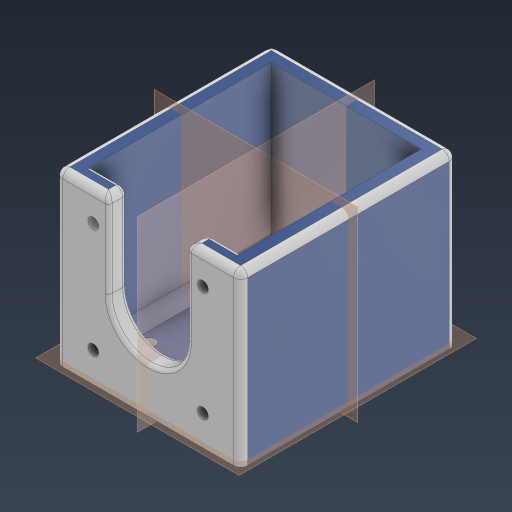
# Autodesk Inventor part: Крепление_мотора
Saved by Autodesk Inventor 2023.2 (Build 272271030, 271C)
## iProperties
Created: 2025-12-13
Part Number: Крепление_мотора
Material: Типовые
Document SubType Name: Modeling
Designer: Олег Коноваленко
Density: 1 g/cm^3
Appearance: По умолчанию
Author: Олег Коноваленко
Autodesk Inventor part; units mm, degrees
sketch "Эскиз1" plane through (0, 0, 0) normal (0, 1, 0) x (-1, 0, 0)
  line L0 (21.15, 25.5) -> (-21.15, 25.5)
  line L1 (-21.15, 25.5) -> (-21.15, -25.5)
  line L2 (-21.15, -25.5) -> (21.15, -25.5)
  line L3 (21.15, -25.5) -> (21.15, 25.5)
  line L4 (21.15, 25.5) -> (-21.15, -25.5) construction
  line L5 (-21.15, 25.5) -> (21.15, -25.5) construction
  point P0 (0, 0)
  dimension "d2" = 51
  dimension "d3" = 42.3
  constraints: 12 end point, 2 midpoint, 2 parallel, 1 horizontal, 1 perpendicular
  measures "d2" distance of L0.end L1.end
  measures "d3" distance of L1.end L2.end
extrude "Выдавливание1" add sketch "Эскиз1" along normal mid plane 2.85
sketch "Эскиз2" plane through (0, 1.425, 0) normal (0, 1, 0) x (1, 0, 0)
  line L0 (-21.15, -25.5) -> (-21.15, 25.5) projected
  line L1 (-21.15, 25.5) -> (-26.15, 25.5)
  line L2 (-26.15, 25.5) -> (-26.15, -25.5)
  line L3 (-26.15, -25.5) -> (-21.15, -25.5)
  line L4 (-21.15, -25.5) -> (-21.15, 25.5)
  point P0 (0, 0)
  dimension "d4" = 5
  constraints: 8 end point, 2 parallel, 1 horizontal, 1 perpendicular, 1 point on line
  measures "d4" distance of L0.end L1.end
extrude "Выдавливание2" add sketch "Эскиз2" along normal blind 45.15 and the other way blind 2.85
mirror "Зеркальное отражение1" about plane through (0, 0, 0) normal (1, 0, 0) of "Выдавливание2"
chamfer "Фаска1" distance 3.2 angle 45 2 edges at (-21.15, 1.425, 0) (21.15, 1.425, 0)
sketch "Эскиз3" plane through (0, 1.425, 0) normal (0, 1, 0) x (1, 0, 0)
  line L0 (-26.15, 25.5) -> (26.15, 25.5) projected
  line L1 (-26.15, 25.5) -> (26.15, 25.5)
  line L2 (26.15, 25.5) -> (26.15, 30.5)
  line L3 (26.15, 30.5) -> (-26.15, 30.5)
  line L4 (-26.15, 30.5) -> (-26.15, 25.5)
  point P0 (0, 0)
  dimension "d17" = 5
  constraints: 8 end point, 2 parallel, 1 horizontal, 1 perpendicular, 1 point on line
  measures "d17" distance of L3.end L0.start
extrude "Выдавливание3" add sketch "Эскиз3" along normal blind 45.15 and the other way blind 2.85
mirror "Зеркальное отражение2" about plane through (0, 0, 0) normal (0, 0, 1) of "Выдавливание3"
sketch "Эскиз7" plane through (-26.15, -1.425, 30.5) normal (0, 0, 1) x (1, 0, 0)
  circle A0 centre (26.15, 24) radius 11 projected
  circle A1 centre (26.15, 24) radius 11.2
  point P0 (26.15, 1.425)
  dimension "d22" = 22.4
  constraints: 1 centre point, 1 coincident
  measures "d22" diameter of A1
extrude "Выдавливание5" cut sketch "Эскиз7" against normal up to next contours A0 | A1
sketch "Эскиз8" plane through (-26.15, -1.425, 30.5) normal (0, 0, 1) x (1, 0, 0)
  circle A0 centre (26.15, 24) radius 11.2 projected
  line L0 (14.95, 24) -> (14.95, 48)
  line L1 (5, 48) -> (47.3, 48) projected
  line L2 (37.35, 24) -> (37.35, 48.1316)
  point P0 (26.15, 1.425)
  point P1 (37.35, 48)
  dimension "d23" = 22.4
  constraints: 4 end point, 2 perpendicular, 2 point on circle, 1 point on line
  measures "d23" distance between parallel lines of L2 L0
extrude "Выдавливание6" cut sketch "Эскиз8" against normal up to next contours A0 L0 L1 L2
fillet "Сопряжение1" radius 2 11 edges at (-11.2, 46.575, 28) (11.2, 46.575, 28) (-26.15, 46.575, 0) (-18.675, 46.575, 30.5) (18.675, 46.575, 30.5) (26.15, 46.575, 0) (0, 46.575, -30.5) (26.15, 22.575, 30.5) (-26.15, 22.575, 30.5) (-26.15, 22.575, -30.5) (26.15, 22.575, -30.5)
fillet "Сопряжение2" radius 1 12 edges at (0, 11.375, 25.5) (11.2, 33.575, 25.5) (11.7858, 45.9892, 25.5) (17.175, 46.575, 25.5) (-11.7858, 45.9892, 25.5) (-17.175, 46.575, 25.5) (-11.2, 33.575, 25.5) (-11.7858, 45.9892, 29.9142) (0, 11.375, 30.5) (11.2, 33.575, 30.5) (11.7858, 45.9892, 29.9142) (-11.2, 33.575, 30.5)
sketch "Эскиз9" plane through (-24.15, -1.425, 30.5) normal (0, 0, 1) x (1, 0, 0)
  circle A0 centre (8.65, 39.5) radius 1.5
  circle A1 centre (39.65, 39.5) radius 1.5
  circle A2 centre (39.65, 8.5) radius 1.5
  circle A3 centre (8.65, 8.5) radius 1.5
  line L0 (8.65, 39.5) -> (39.65, 39.5) construction
  line L1 (39.65, 39.5) -> (39.65, 8.5) construction
  line L2 (39.65, 8.5) -> (8.65, 8.5) construction
  line L3 (8.65, 8.5) -> (8.65, 39.5) construction
  arc A4 (12.95, 24) -> (35.35, 24) centre (24.15, 24) ccw projected
  line L4 (8.65, 39.5) -> (39.65, 8.5) construction
  line L5 (39.65, 39.5) -> (8.65, 8.5) construction
  line L6 (24.15, 62.1506) -> (24.15, -10.3584) projected
  point P0 (24.15, 1.425)
  point P1 (24.15, 24)
  point P2 (24.15, 24)
  dimension "d28" = 3
  dimension "d29" = 31
  constraints: 12 end point, 4 centre point, 4 perpendicular, 3 equal radius, 2 midpoint, 1 coincident, 1 horizontal, 1 parallel, 1 point on line
  measures "d28" diameter of A0
  measures "d29" distance of L0.start L0.end
extrude "Выдавливание7" cut sketch "Эскиз9" against normal up to next
sketch "Эскиз10" plane through (0, -1.425, 0) normal (0, -1, 0) x (1, 0, 0)
  line L0 (15, -15) -> (-15, -15) construction
  line L1 (-15, -15) -> (-15, 15) construction
  line L2 (-15, 15) -> (15, 15) construction
  line L3 (15, 15) -> (15, -15) construction
  line L4 (15, -15) -> (-15, 15) construction
  line L5 (-15, -15) -> (15, 15) construction
  circle A0 centre (-15, -15) radius 1.6
  circle A1 centre (-15, 15) radius 1.6
  circle A2 centre (15, -15) radius 1.6
  circle A3 centre (15, 15) radius 1.6
  point P0 (0, 0)
  dimension "d32" = 30
  dimension "d33" = 3.2
  constraints: 12 end point, 4 centre point, 3 coincident, 3 equal radius, 2 midpoint, 2 parallel, 2 perpendicular, 1 horizontal
  measures "d32" distance of L0.start L0.end
  measures "d33" diameter of A0
extrude "Выдавливание8" cut sketch "Эскиз10" against normal up to next
